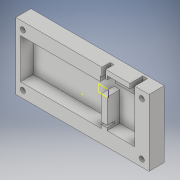
# Autodesk Inventor part: ArduinPanel2
Saved by Autodesk Inventor 2018 (Build 220112000, 112)
## iProperties
Created: 2020-03-31
Part Number: ArduinPanel2
Material: Generic
Document SubType Name: Modeling
Designer: emile
Density: 1 g/cm^3
Appearance: Default
Mass: 177.496 g
Surface Area: 535.214 cm^2
Volume: 177.496 cm^3
Author: emile
Autodesk Inventor part; units mm, degrees
ref_plane "YZ Plane" through (0, 0, 0) normal (1, 0, 0) x (0, 1, 0)
ref_plane "XZ Plane" through (0, 0, 0) normal (0, 1, 0) x (-1, 0, 0)
ref_plane "XY Plane" through (0, 0, 0) normal (0, 0, 1) x (1, 0, 0)
sketch "Sketch1" plane through (0, 0, 0) normal (0, 0, 1) x (1, 0, 0)
  line L0 (88.9, -44.45) -> (-88.9, -44.45)
  line L1 (-88.9, -44.45) -> (-88.9, 44.45)
  line L2 (-88.9, 44.45) -> (88.9, 44.45)
  line L3 (88.9, 44.45) -> (88.9, -44.45)
  line L4 (88.9, -44.45) -> (-88.9, 44.45) construction
  line L5 (-88.9, -44.45) -> (88.9, 44.45) construction
  line L6 (25.4, -26.7335) -> (-82.55, -26.7335)
  line L7 (-82.55, -26.7335) -> (-82.55, 26.7335)
  line L8 (-82.55, 26.7335) -> (25.4, 26.7335)
  line L9 (25.4, 26.7335) -> (25.4, -26.7335)
  line L10 (25.4, -26.7335) -> (-82.55, 26.7335) construction
  line L11 (-82.55, -26.7335) -> (25.4, 26.7335) construction
  line L12 (34.29, 23.1775) -> (20.955, 23.1775)
  line L13 (20.955, 23.1775) -> (20.955, 13.5255)
  line L14 (20.955, 13.5255) -> (34.29, 13.5255)
  line L15 (34.29, 13.5255) -> (34.29, 23.1775)
  line L16 (34.29, 23.1775) -> (20.955, 13.5255) construction
  line L17 (20.955, 23.1775) -> (34.29, 13.5255) construction
  line L18 (23.8125, 33.3375) -> (26.162, 33.3375)
  line L19 (26.162, 33.3375) -> (26.162, 44.45)
  line L20 (31.242, 44.45) -> (31.242, 33.3375)
  line L21 (31.242, 33.3375) -> (34.29, 33.3375)
  line L22 (34.29, 33.3375) -> (34.29, 23.1775)
  line L23 (26.162, 33.3375) -> (31.242, 33.3375) construction
  line L24 (26.162, 44.45) -> (31.242, 44.45)
  line L25 (25.4, 23.1775) -> (34.29, 23.1775)
  line L26 (25.4, 23.1775) -> (25.4, 26.7335)
  line L27 (25.4, 26.7335) -> (25.4, 26.7335)
  line L28 (23.8125, 33.3375) -> (23.8125, 26.7335)
  point P0 (0, 0)
  point P1 (-28.575, 0)
  point P2 (-28.575, 0)
  point P3 (0, 0)
  point P4 (27.6225, 18.3515)
  point P5 (28.702, 33.3375)
  dimension "d0" = 177.8
  dimension "d1" = 88.9
  dimension "d2" = 107.95
  dimension "d3" = 53.467
  dimension "d4" = 6.35
  dimension "d5" = 103.505
  dimension "d7" = 8.382
  dimension "d8" = 9.652
  dimension "d13" = 13.335
  dimension "d15" = 5.08
  dimension "d17" = 10.16
  dimension "d24" = 1.5875
  dimension "d25" = 5.588
  constraints: 58 end point, 9 midpoint, 8 perpendicular, 6 parallel, 6 point on line, 3 collinear, 3 horizontal, 2 vertical, 1 horizontal alignment
  measures "d0" distance of L1.end L2.end
  measures "d1" distance of L0.end L1.end
  measures "d2" distance of L7.end L8.end
  measures "d3" distance between parallel lines of L6 L8
  measures "d4" distance between parallel lines of L1 L7
  measures "d5" distance between parallel lines of L7 L13
  measures "d7" distance from line of L8 point (27.622, 18.351)
  measures "d8" distance of L14.end L12.start
  measures "d13" distance of L12.start L12.end
  measures "d15" distance between parallel lines of L19 L20
  measures "d17" distance between parallel lines of L12 L21
  measures "d24" distance between parallel lines of L9 L28
  measures "d25" distance from line of L22 point (28.702, 33.338)
extrude "Extrusion1" add sketch "Sketch1" along normal blind 17.145
extrude "Extrusion2" cut sketch "Sketch1" along normal through all contours L20 L21 L22 L12 L9 L8 L28 L18 L19 L2
sketch "Sketch3" plane through (0, 0, 0) normal (0, 0, -1) x (-1, 0, 0)
  line L0 (-31.242, 33.3375) -> (-31.242, 44.45) projected
  line L1 (-31.242, 44.45) -> (-88.9, 44.45) projected
  line L2 (-88.9, 44.45) -> (-88.9, -44.45) projected
  line L3 (-88.9, -44.45) -> (88.9, -44.45) projected
  line L4 (88.9, -44.45) -> (88.9, 44.45) projected
  line L5 (88.9, 44.45) -> (-26.162, 44.45) projected
  line L6 (-26.162, 44.45) -> (-26.162, 33.3375) projected
  line L7 (-26.162, 33.3375) -> (-23.8125, 33.3375) projected
  line L8 (-34.29, 23.1775) -> (-34.29, 33.3375) projected
  line L9 (-34.29, 33.3375) -> (-31.242, 33.3375) projected
  line L10 (-26.162, 44.45) -> (88.9, 44.45) projected
  line L11 (-26.162, 44.45) -> (-31.242, 44.45)
  line L12 (-23.8125, 33.3375) -> (-23.8125, 26.7335) projected
  line L13 (-23.8125, 26.7335) -> (-25.4, 26.7335) projected
  line L14 (-25.4, 26.7335) -> (-25.4, 23.1775) projected
  line L15 (-25.4, 23.1775) -> (-34.29, 23.1775) projected
  point P0 (0, 0)
  constraints: 2 end point, 1 collinear
extrude "Extrusion4" add sketch "Sketch3" along normal blind 3.175
ref_plane "Work Plane1" through (-28.575, -26.7335, 12.7) normal (1, 0, 0) x (0, 0, -1)
ref_plane "Work Plane2" through (-82.55, 0, 12.7) normal (0, -1, 0) x (1, 0, 0)
sketch "Sketch5" plane through (0, 0, 17.145) normal (0, 0, 1) x (1, 0, 0)
  line L0 (69.85, -25.4) -> (33.02, -25.4)
  line L1 (33.02, -25.4) -> (33.02, 25.4)
  line L2 (33.02, 25.4) -> (69.85, 25.4)
  line L3 (69.85, 25.4) -> (69.85, -25.4)
  line L4 (69.85, -25.4) -> (33.02, 25.4) construction
  line L5 (33.02, -25.4) -> (69.85, 25.4) construction
  line L6 (124.46, 0) -> (-124.46, 0) projected
  line L7 (88.9, -44.45) -> (88.9, 44.45) projected
  line L8 (69.85, 25.4) -> (63.5, 25.4)
  line L9 (63.5, 25.4) -> (63.5, 44.45)
  line L10 (63.5, 44.45) -> (69.85, 44.45)
  line L11 (69.85, 44.45) -> (69.85, 25.4)
  line L12 (88.9, 44.45) -> (-88.9, 44.45) projected
  point P0 (0, 0)
  point P1 (51.435, 0)
  point P2 (51.435, 0)
  point P3 (31.242, 44.45)
  dimension "d26" = 36.83
  dimension "d27" = 50.8
  dimension "d28" = 19.05
  dimension "d29" = 6.35
  constraints: 20 end point, 4 parallel, 3 midpoint, 3 point on line, 2 perpendicular, 1 horizontal
  measures "d26" distance of L1.end L2.end
  measures "d27" distance of L2.end L0.start
  measures "d28" distance between parallel lines of L7 L3
  measures "d29" distance between parallel lines of L11 L9
extrude "Extrusion5" cut sketch "Sketch5" against normal up to surface (17.145 mm away) contours L0 L1 L6 L3 | L6 L1 L2 L3 | L2 L9 L10 L11
ref_plane "Work Plane3" through (51.435, -25.4, 17.145) normal (1, 0, 0) x (0, 0, -1)
ref_plane "Work Plane4" through (33.02, 0, 17.145) normal (0, -1, 0) x (1, 0, 0)
sketch "Sketch6" plane through (0, 0, 17.145) normal (0, 0, 1) x (1, 0, 0)
  line L0 (69.85, 44.45) -> (69.85, -25.4) projected
  line L1 (69.85, -25.4) -> (33.02, -25.4) projected
  line L2 (33.02, -25.4) -> (33.02, 23.1775) projected
  line L3 (34.29, 25.4) -> (63.5, 25.4) projected
  line L4 (63.5, 25.4) -> (63.5, 44.45) projected
  line L5 (26.162, 44.45) -> (-88.9, 44.45) projected
  line L6 (-88.9, 44.45) -> (-88.9, -44.45) projected
  line L7 (-88.9, -44.45) -> (88.9, -44.45) projected
  line L8 (88.9, -44.45) -> (88.9, 44.45) projected
  line L9 (88.9, 44.45) -> (69.85, 44.45) projected
  line L10 (33.02, -25.4) -> (33.02, 25.4) projected
  line L11 (39.37, 25.4) -> (63.5, 25.4)
  line L12 (63.5, 25.4) -> (63.5, 38.1)
  line L13 (63.5, 38.1) -> (39.37, 38.1)
  line L14 (39.37, 38.1) -> (39.37, 25.4)
  line L15 (39.37, 38.1) -> (33.02, 38.1)
  line L16 (33.02, 38.1) -> (33.02, 25.4)
  line L17 (33.02, 25.4) -> (39.37, 25.4)
  line L18 (36.195, 25.4) -> (36.195, -22.225)
  line L19 (33.02, 25.4) -> (33.02, -19.05)
  line L20 (33.02, -19.05) -> (25.4, -19.05)
  line L21 (25.4, -26.7335) -> (25.4, 13.5255) projected
  line L22 (36.195, -22.225) -> (25.4, -22.225)
  line L23 (25.4, -19.05) -> (25.4, -22.225)
  line L24 (63.5, 44.45) -> (31.242, 44.45) projected
  line L25 (31.242, 44.45) -> (31.242, 33.3375) projected
  line L26 (31.242, 33.3375) -> (34.29, 33.3375) projected
  line L27 (34.29, 33.3375) -> (34.29, 25.4) projected
  line L28 (33.02, 23.1775) -> (25.4, 23.1775) projected
  line L29 (25.4, 23.1775) -> (25.4, 26.7335) projected
  line L30 (25.4, 26.7335) -> (23.8125, 26.7335) projected
  line L31 (23.8125, 26.7335) -> (23.8125, 33.3375) projected
  line L32 (23.8125, 33.3375) -> (26.162, 33.3375) projected
  line L33 (26.162, 33.3375) -> (26.162, 44.45) projected
  point P0 (0, 0)
  dimension "d32" = 12.7
  dimension "d33" = 3.175
  dimension "d34" = 3.175
  dimension "d35" = 22.225
  constraints: 24 end point, 5 perpendicular, 2 parallel, 2 point on line, 2 vertical, 1 collinear, 1 horizontal, 1 midpoint
  measures "d32" distance between parallel lines of L3 L13
  measures "d33" distance between parallel lines of L19 L18
  measures "d34" distance between parallel lines of L22 L20
  measures "d35" distance between parallel lines of L7 L22
extrude "Extrusion6" cut sketch "Sketch6" against normal blind 9.525 contours L14 L13 L4 L3
extrude "Extrusion7" cut sketch "Sketch6" against normal blind 9.525 contours L22 L21 L20 L2 | L2 L10 L17 L3 L18 L22 | L3 L27 L26 L16 L15 L14 | L16 L26 L27 L17
sketch "Sketch7" plane through (0, 0, 0) normal (0, 0, 1) x (1, 0, 0)
  line L0 (26.162, 44.45) -> (26.162, 33.3375) projected
  line L1 (26.162, 33.3375) -> (23.8125, 33.3375) projected
  line L2 (23.8125, 33.3375) -> (23.8125, 26.7335) projected
  line L3 (34.29, 25.4) -> (34.29, 33.3375) projected
  line L4 (34.29, 33.3375) -> (31.242, 33.3375) projected
  line L5 (31.242, 33.3375) -> (31.242, 44.45) projected
  line L6 (26.162, 44.45) -> (31.242, 44.45) projected
  line L7 (26.162, 33.3375) -> (26.162, 44.45) projected
  line L8 (26.162, 33.3375) -> (31.242, 33.3375)
  line L9 (23.8125, 26.7335) -> (25.4, 26.7335) projected
  line L10 (25.4, 26.7335) -> (25.4, 23.1775) projected
  line L11 (25.4, 23.1775) -> (33.02, 23.1775) projected
  line L12 (33.02, -25.4) -> (33.02, 23.1775) projected
  line L13 (69.85, -25.4) -> (33.02, -25.4) projected
  line L14 (69.85, 44.45) -> (69.85, -25.4) projected
  line L15 (63.5, 44.45) -> (69.85, 44.45) projected
  line L16 (63.5, 25.4) -> (63.5, 44.45) projected
  line L17 (34.29, 25.4) -> (63.5, 25.4) projected
  point P0 (0, 0)
  constraints: 2 end point, 1 perpendicular
extrude "Extrusion8" add sketch "Sketch7" along normal blind 6.35 contours L6 L5 L8 L0
extrude "Extrusion9" cut sketch "Sketch1" along normal through all contours L8 L9 L12 L13 L14 L6 L7 | L9 L14 L13 L12
sketch "Sketch8" plane through (0, 0, 17.145) normal (0, 0, 1) x (1, 0, 0)
  line L0 (20.955, 13.5255) -> (34.29, 13.5255) projected
  line L1 (20.955, 23.1775) -> (20.955, 13.5255) projected
  line L2 (34.29, 23.1775) -> (20.955, 23.1775) projected
  line L3 (34.29, 13.5255) -> (34.29, 23.1775)
  point P0 (0, 0)
  constraints: 2 end point, 1 vertical
extrude "Extrusion10" cut sketch "Sketch8" against normal up to surface (17.145 mm away)
sketch "Sketch9" plane through (0, 0, -3.175) normal (0, 0, -1) x (-1, 0, 0)
  point P0 (-79.375, 34.925)
  point P1 (79.375, 34.925)
  point P2 (79.375, -34.925)
  point P3 (-79.375, -34.925)
hole "Hole1" at (79.375, 34.925, -3.175) at (-79.375, 34.925, -3.175) at (-79.375, -34.925, -3.175) at (79.375, -34.925, -3.175) direction (0, 0, 1) diameter 6.7564 depth 3.175
sketch "Sketch10" plane through (0, 0, -3.175) normal (0, 0, -1) x (-1, 0, 0)
  circle A0 centre (79.375, -34.925) radius 3.3782 projected
  circle A1 centre (-79.375, 34.925) radius 3.3782 projected
  circle A2 centre (79.375, 34.925) radius 3.3782 projected
  circle A3 centre (-79.375, -34.925) radius 3.3782 projected
  line L0 (88.9, 44.45) -> (-88.9, 44.45) projected
  line L1 (-88.9, 44.45) -> (-88.9, -44.45) projected
  line L2 (-88.9, -44.45) -> (88.9, -44.45) projected
  line L3 (88.9, -44.45) -> (88.9, 44.45) projected
  point P0 (0, 0)
extrude "Extrusion11" cut sketch "Sketch10" against normal through all contours A0 | A1 | A2 | A3
equation "\"d34\" = d33"
body "Solid1"
